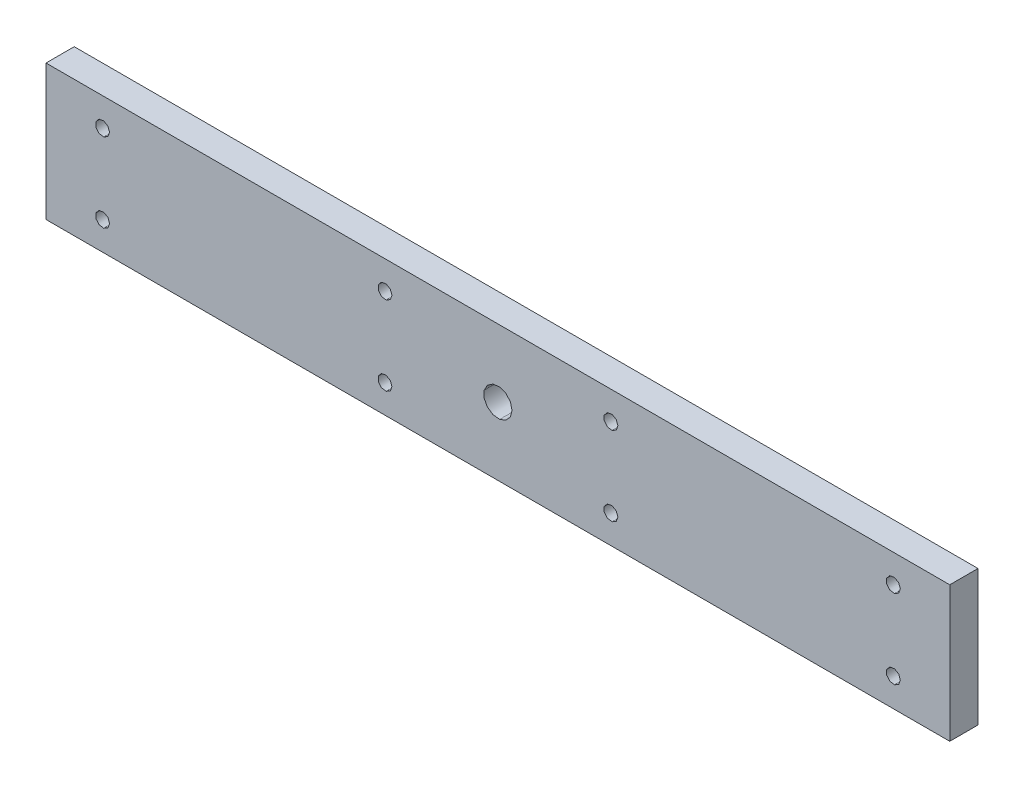
# Autodesk Inventor part: arm
Saved by Autodesk Inventor 2023 (Build 270158000, 158)
## iProperties
Created: 2023-10-16
Part Number: arm
Material: Generic
Document SubType Name: Modeling
Designer: Nate
Density: 1 g/cm^3
Appearance: Default
Author: Nate
Autodesk Inventor part; units mm, degrees
ref_plane "YZ Plane" through (0, 0, 0) normal (1, 0, 0) x (0, 1, 0)
ref_plane "XZ Plane" through (0, 0, 0) normal (0, 1, 0) x (-1, 0, 0)
ref_plane "XY Plane" through (0, 0, 0) normal (0, 0, 1) x (1, 0, 0)
sketch "Sketch1" plane through (0, 0, 0) normal (0, 0, 1) x (1, 0, 0)
  line L0 (0, 0) -> (150, 0)
  line L1 (150, 0) -> (150, 38.1)
  line L2 (150, 38.1) -> (0, 38.1)
  line L3 (0, 38.1) -> (0, 0)
  line L4 (0, 0) -> (-549.9999, 0)
  line L5 (-549.9999, 0) -> (-549.9999, 38.1)
  line L6 (-549.9999, 38.1) -> (0, 38.1)
  line L7 (0, 38.1) -> (0, 0)
  circle A0 centre (0, 19.05) radius 3.175
  circle A1 centre (137.3, 19.05) radius 3.175
  circle A2 centre (-537.2999, 25.4) radius 3.175
  circle A3 centre (-499.1999, 12.7) radius 3.175
  line L8 (-101.6, 34.29) -> (101.6, 34.29)
  line L9 (101.6, 34.29) -> (101.6, 3.81)
  line L10 (101.6, 3.81) -> (-101.6, 3.81)
  line L11 (-101.6, 3.81) -> (-101.6, 34.29)
  circle A4 centre (-88.9, 27.94) radius 1.5875
  circle A5 centre (-88.9, 10.16) radius 1.5875
  circle A6 centre (-25.4, 10.16) radius 1.5875
  circle A7 centre (-25.4, 27.94) radius 1.5875
  circle A8 centre (25.4, 27.94) radius 1.5875
  circle A9 centre (25.4, 10.16) radius 1.5875
  circle A10 centre (88.9, 10.16) radius 1.5875
  circle A11 centre (88.9, 27.94) radius 1.5875
  point P0 (150, 19.05)
  point P1 (-101.6, 19.05)
  point P2 (0, 15.875)
  point P3 (0, 22.225)
  dimension "d0" = 150
  dimension "d1" = 38.1
  dimension "d2" = 38.1
  dimension "d3" = 549.9999
  dimension "d4" = 6.35
  dimension "d5" = 6.35
  dimension "d6" = 6.35
  dimension "d7" = 6.35
  dimension "d8" = 12.7
  dimension "d9" = 12.7
  dimension "d10" = 12.7
  dimension "d11" = 50.8
  dimension "d12" = 19.05
  dimension "d13" = 12.7
  dimension "d14" = 203.2
  dimension "d15" = 3.81
  dimension "d16" = 3.81
  dimension "d17" = 101.6
  dimension "d18" = 3.175
  dimension "d19" = 3.175
  dimension "d20" = 3.175
  dimension "d21" = 3.175
  dimension "d22" = 3.175
  dimension "d23" = 3.175
  dimension "d24" = 3.175
  dimension "d25" = 3.175
  dimension "d26" = 6.35
  dimension "d27" = 6.35
  dimension "d28" = 6.35
  dimension "d29" = 6.35
  dimension "d30" = 6.35
  dimension "d31" = 6.35
  dimension "d32" = 12.7
  dimension "d33" = 12.7
  dimension "d34" = 12.7
  dimension "d35" = 12.7
  dimension "d36" = 25.4
  dimension "d37" = 25.4
  dimension "d38" = 25.4
  dimension "d39" = 25.4
  dimension "d40" = 6.35
  dimension "d41" = 6.35
  constraints: 24 end point, 12 centre point, 6 parallel, 3 horizontal, 3 midpoint, 3 perpendicular, 1 coincident
  measures "d0" distance from line of L1 point (0, 19.05)
  measures "d1" distance between parallel lines of L2 L0
  measures "d2" distance between parallel lines of L6 L4
  measures "d3" distance between parallel lines of L5 L3
  measures "d4" diameter of A0
  measures "d5" diameter of A1
  measures "d6" diameter of A2
  measures "d7" diameter of A3
  measures "d8" distance from line of A3.centre L4
  measures "d9" distance from line of L6 A2.centre
  measures "d10" distance from line of A2.centre L5
  measures "d11" distance from line of L5 A3.centre
  measures "d12" distance from line of A1.centre L0
  measures "d13" distance of point (150, 19.05) A1.centre
  measures "d14" distance of L9.end L10.end
  measures "d15" distance between parallel lines of L6 L8
  measures "d16" distance between parallel lines of L4 L10
  measures "d17" distance of point (-101.6, 19.05) point (0, 19.05)
  measures "d18" diameter of A4
  measures "d19" diameter of A5
  measures "d20" diameter of A6
  measures "d21" diameter of A7
  measures "d22" diameter of A8
  measures "d23" diameter of A9
  measures "d24" diameter of A10
  measures "d25" diameter of A11
  measures "d26" distance from line of L8 A4.centre
  measures "d27" distance from line of L10 A5.centre
  measures "d28" distance from line of A6.centre L10
  measures "d29" distance from line of L8 A7.centre
  measures "d30" distance from line of L8 A11.centre
  measures "d31" distance from line of A10.centre L10
  measures "d32" distance from line of L9 A10.centre
  measures "d33" distance from line of L9 A11.centre
  measures "d34" distance from line of L11 A5.centre
  measures "d35" distance from line of L11 A4.centre
  measures "d36" distance from line of L3 A6.centre
  measures "d37" distance from line of L3 A7.centre
  measures "d38" distance from line of A8.centre L3
  measures "d39" distance from line of A9.centre L3
  measures "d40" distance from line of L8 A8.centre
  measures "d41" distance from line of L10 A9.centre
extrude "Extrusion1" add sketch "Sketch1" along normal blind 6.35 contours L10 L11 L8 L3 A0 | L3 A0 L8 L9 L10
body "Solid1"
